Autodesk Fusion 360 part; units mm, degrees
(part 4 of 5)
sketch "Sketch14" plane through (0, -22.5, 0) normal (0, -1, 0) x (1, 0, 0)
  line L0 (26.575, -10) -> (26.575, 1)
  line L1 (26.575, 1) -> (-26.575, 1)
  line L2 (-26.575, 1) -> (-26.575, -10)
  line L3 (-26.575, -10) -> (26.575, -10)
  line L4 (-15.5, -1.5) -> (15.5, -1.5)
  line L5 (17.5, -3.5) -> (17.5, -5.5)
  line L6 (15.5, -7.5) -> (-15.5, -7.5)
  line L7 (-17.5, -5.5) -> (-17.5, -3.5)
  arc A0 (-15.5, -1.5) -> (-17.5, -3.5) centre (-15.5, -3.5) ccw
  arc A1 (-17.5, -5.5) -> (-15.5, -7.5) centre (-15.5, -5.5) ccw
  arc A2 (15.5, -7.5) -> (17.5, -5.5) centre (15.5, -5.5) ccw
  arc A3 (17.5, -3.5) -> (15.5, -1.5) centre (15.5, -3.5) ccw
  dimension "d131" = 2.5
  dimension "d132" = 2.5
  dimension "d133" = 9.075
  dimension "d134" = 9.075
  dimension "d135" = 2
  constraint horizontal L4
  constraint vertical L5
  constraint horizontal L6
  constraint vertical L7
  constraint tangent L4 A0
  constraint tangent L7 A0
  constraint tangent L7 A1
  constraint tangent L6 A1
  constraint equal A0 A1
  constraint tangent L6 A2
  constraint tangent L5 A2
  constraint equal A0 A2
  constraint tangent L4 A3
  constraint tangent L5 A3
  constraint equal A0 A3
  measures "d131" distance of L1 L4
  measures "d132" distance of L3 L6
  measures "d133" distance of L2 L7
  measures "d134" distance of L0 L5
  measures "d135" radius of A0
extrude "Extrude16" cut sketch "Sketch14" against normal blind 4 contours L4 L5 L6 L7 A0 A1 A2 A3 bodies 1
sketch "Sketch15" plane through (-26.575, 0, 0) normal (-1, 0, 0) x (0, -1, 0)
  line L0 (-22.5, 38.5) -> (-28.5, 38.5)
  line L1 (-28.5, 38.5) -> (-28.5, -10)
  line L2 (-28.5, -10) -> (22.5, -10)
  line L3 (22.5, -10) -> (22.5, 1)
  line L4 (22.5, 1) -> (-22.5, 1)
  line L5 (-22.5, 1) -> (-22.5, 38.5)
  line L6 (-13, -1.5) -> (13, -1.5)
  line L7 (15, -3.5) -> (15, -5.5)
  line L8 (13, -7.5) -> (-13, -7.5)
  line L9 (-15, -5.5) -> (-15, -3.5)
  arc A0 (15, -3.5) -> (13, -1.5) centre (13, -3.5) ccw
  arc A1 (13, -7.5) -> (15, -5.5) centre (13, -5.5) ccw
  arc A2 (-15, -5.5) -> (-13, -7.5) centre (-13, -5.5) ccw
  arc A3 (-13, -1.5) -> (-15, -3.5) centre (-13, -3.5) ccw
  dimension "d138" = 2.5
  dimension "d139" = 2.5
  dimension "d140" = 7.5
  dimension "d141" = 13.5
  dimension "d142" = 2
  constraint horizontal L6
  constraint vertical L7
  constraint horizontal L8
  constraint vertical L9
  constraint tangent L7 A0
  constraint tangent L6 A0
  constraint tangent L7 A1
  constraint tangent L8 A1
  constraint equal A0 A1
  constraint tangent L8 A2
  constraint tangent L9 A2
  constraint equal A0 A2
  constraint tangent L9 A3
  constraint tangent L6 A3
  constraint equal A0 A3
  measures "d138" distance of L4 L6
  measures "d139" distance of L2 L8
  measures "d140" distance of L3 L7
  measures "d141" distance of L1 L9
  measures "d142" radius of A0
extrude "Extrude17" cut sketch "Sketch15" against normal blind 4 contours L6 L7 L8 L9 A0 A1 A2 A3 bodies 1
sketch "Sketch16" plane through (0, 28.5, 0) normal (0, 1, 0) x (-1, 0, 0)
  line L0 (-24.075, 6) -> (-24.075, 7)
  arc A0 (-21.575, 9.5) -> (-24.075, 7) centre (-21.575, 7) ccw
  line L1 (-21.575, 9.5) -> (21.575, 9.5)
  arc A1 (24.075, 7) -> (21.575, 9.5) centre (21.575, 7) ccw
  line L2 (24.075, 7) -> (24.075, 6)
  arc A2 (21.575, 3.5) -> (24.075, 6) centre (21.575, 6) ccw
  line L3 (21.575, 3.5) -> (-21.575, 3.5)
  arc A3 (-24.075, 6) -> (-21.575, 3.5) centre (-21.575, 6) ccw
  circle A4 centre (0, 24.5) radius 12.5
  line L4 (26.575, 38.5) -> (-26.575, 38.5)
  line L5 (-26.575, 38.5) -> (-26.575, -10)
  line L6 (-26.575, -10) -> (26.575, -10)
  line L7 (26.575, -10) -> (26.575, 38.5)
  circle A5 centre (20, 18.5) radius 5
  circle A6 centre (-20, 30.5) radius 5
  circle A7 centre (20, 30.5) radius 5
  circle A8 centre (-20, 18.5) radius 5
  line L8 (-15.5, -1.5) -> (15.5, -1.5)
  line L9 (17.5, -3.5) -> (17.5, -5.5)
  line L10 (15.5, -7.5) -> (-15.5, -7.5)
  line L11 (-17.5, -5.5) -> (-17.5, -3.5)
  arc A9 (-15.5, -1.5) -> (-17.5, -3.5) centre (-15.5, -3.5) ccw
  arc A10 (-17.5, -5.5) -> (-15.5, -7.5) centre (-15.5, -5.5) ccw
  arc A11 (15.5, -7.5) -> (17.5, -5.5) centre (15.5, -5.5) ccw
  arc A12 (17.5, -3.5) -> (15.5, -1.5) centre (15.5, -3.5) ccw
  dimension "d145" = 5
  dimension "d146" = 2.5
  dimension "d147" = 9.075
  dimension "d148" = 9.075
  dimension "d149" = 2
  constraint horizontal L8
  constraint vertical L9
  constraint horizontal L10
  constraint vertical L11
  constraint tangent L8 A9
  constraint tangent L11 A9
  constraint tangent L11 A10
  constraint tangent L10 A10
  constraint equal A9 A10
  constraint tangent L10 A11
  constraint tangent L9 A11
  constraint equal A9 A11
  constraint tangent L9 A12
  constraint tangent L8 A12
  constraint equal A9 A12
  measures "d145" distance of L3 L8
  measures "d146" distance of L6 L10
  measures "d147" distance of L5 L11
  measures "d148" distance of L7 L9
  measures "d149" radius of A9
extrude "Extrude18" cut sketch "Sketch16" against normal blind 10 contours L8 L9 L10 L11 A9 A10 A11 A12 bodies 1
equation "d7 = ( 2.25 in / 2 )"
equation "d8 = ( 45 / 2 ) * 1 mm"
equation "d31 = ( 2.25 in - 40 mm ) / 2"
equation "d127 = 7.5 mm + 6 mm"
equation "d133 = ( ( 53.15 - 35 ) / 2 ) * 1 mm"
equation "d134 = ( ( 53.15 - 35 ) / 2 ) * 1 mm"

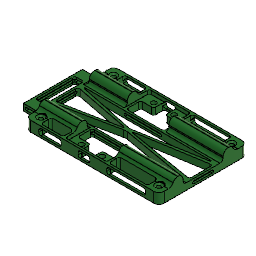
design "TM Foundation"
Autodesk Fusion 360 part; units mm, degrees
sketch "Sketch1" plane through (0, 0, 0) normal (0, 0, 1) x (1, 0, 0)
  line L0 (-72.5, 28.55) -> (72.5, 28.55)
  line L1 (72.5, 28.55) -> (72.5, -28.55)
  line L2 (72.5, -28.55) -> (-72.5, -28.55)
  line L3 (-72.5, -28.55) -> (-72.5, 28.55)
  dimension "d1" = 145
  dimension "d2" = 72.5
  dimension "d3" = 57.1
  dimension "d4" = 28.55
  constraint horizontal L0
  constraint vertical L1
  constraint horizontal L2
  constraint vertical L3
  measures "d1" distance of L1 L3
  measures "d2" distance of origin L1
  measures "d3" distance of L0 L2
  measures "d4" distance of origin L0
extrude "Extrude1" add sketch "Sketch1" along normal blind 6.5
ref_plane "WorkPlane1" through (-62.5, 0, 3.25) normal (-1, 0, 0) x (0, -1, 0)
sketch "Sketch6" plane through (-62.5, 0, 0) normal (-1, 0, 0) x (0, -1, 0)
  line L0 (-28.55, 6.5) -> (-28.55, 15.75)
  line L1 (-28.55, 15.75) -> (-24.3, 15.75)
  line L2 (-16.3, 6.5) -> (16.3, 6.5)
  line L3 (28.55, 6.5) -> (28.55, 15.75)
  line L4 (28.55, 15.75) -> (24.3, 15.75)
  line L5 (-19.3, 10.75) -> (-19.3, 9.5)
  line L6 (19.3, 10.75) -> (19.3, 9.5)
  arc A0 (-19.3, 9.5) -> (-16.3, 6.5) centre (-16.3, 9.5) ccw
  arc A1 (16.3, 6.5) -> (19.3, 9.5) centre (16.3, 9.5) ccw
  arc A2 (-19.3, 10.75) -> (-24.3, 15.75) centre (-24.3, 10.75) ccw
  arc A3 (24.3, 15.75) -> (19.3, 10.75) centre (24.3, 10.75) ccw
  line L7 (-28.55, 6.5) -> (28.55, 6.5)
  point P0 (-19.3, 15.75)
  point P1 (-28.55, 0)
  point P2 (-28.55, 6.5)
  point P3 (-28.55, 6.5)
  point P4 (19.3, 15.75)
  dimension "d36" = 9.25
  dimension "d37" = 9.25
  dimension "d38" = 57.1
  dimension "d39" = 9.25
  dimension "d40" = 9.25
  dimension "d41" = 3
  dimension "d42" = 5
  constraint vertical L0
  constraint perpendicular L0 L1
  constraint vertical P3 P1
  constraint coincident P3 P2
  constraint perpendicular L0 L2
  constraint perpendicular L2 L3
  constraint perpendicular L3 L4
  constraint perpendicular L2 L5
  constraint perpendicular L2 L6
  constraint coincident P3 L2
  constraint tangent L5 A0
  constraint tangent L2 A0
  constraint coincident L3.start L2
  constraint tangent L2 A1
  constraint tangent L6 A1
  constraint equal A0 A1
  constraint coincident P0 L1
  constraint coincident P0 L5
  constraint tangent L1 A2
  constraint tangent L5 A2
  constraint coincident P4 L6
  constraint coincident P4 L4
  constraint tangent L6 A3
  constraint tangent L4 A3
  constraint equal A2 A3
  measures "d36" distance of P3 L0.end
  measures "d37" distance of L0.end P0
  measures "d38" distance of P3 L3.start
  measures "d39" distance of L3.start L3.end
  measures "d40" distance of L3.end P4
  measures "d41" radius of A0
  measures "d42" radius of A2
extrude "Extrude6" add sketch "Sketch6" against normal blind 135
extrude "Extrude7" cut 2 faces at (-62.5, -24.05, 11) (-62.5, 24.05, 11) along direction (1, 0, 0) blind 6
extrude "Extrude12" add 1 faces at (29.5, -28.55, 7.4167) along direction (0, -1, 0) blind 14.05
extrude "Extrude13" add 1 faces at (29.5, 28.55, 7.4167) along direction (0, 1, 0) blind 14.05
sketch "Sketch10" plane through (0, 0, 15.75) normal (0, 0, 1) x (-1, 0, 0)
  line L0 (56.5, 24.3) -> (56.5, 42.6)
  line L1 (56.5, 42.6) -> (-72.5, 42.6)
  line L2 (-72.5, 42.6) -> (-72.5, 24.3)
  line L3 (-72.5, 24.3) -> (56.5, 24.3)
  line L4 (18.05, -40.6) -> (-18.05, -40.6)
  line L5 (-20.05, -38.6) -> (-20.05, 38.6)
  line L6 (-18.05, 40.6) -> (18.05, 40.6)
  line L7 (20.05, 38.6) -> (20.05, -38.6)
  line L8 (56.5, -42.6) -> (-72.5, -42.6)
  arc A0 (20.05, 38.6) -> (18.05, 40.6) centre (18.05, 38.6) ccw
  arc A1 (-18.05, 40.6) -> (-20.05, 38.6) centre (-18.05, 38.6) ccw
  arc A2 (-20.05, -38.6) -> (-18.05, -40.6) centre (-18.05, -38.6) ccw
  arc A3 (18.05, -40.6) -> (20.05, -38.6) centre (18.05, -38.6) ccw
  dimension "d68" = 52.45
  dimension "d69" = 36.45
  dimension "d70" = 2
  dimension "d71" = 2
  dimension "d74" = 2
  constraint horizontal L4
  constraint vertical L5
  constraint horizontal L6
  constraint vertical L7
  constraint tangent L7 A0
  constraint tangent L6 A0
  constraint tangent L6 A1
  constraint tangent L5 A1
  constraint equal A0 A1
  constraint tangent L5 A2
  constraint tangent L4 A2
  constraint equal A0 A2
  constraint tangent L4 A3
  constraint tangent L7 A3
  constraint equal A0 A3
  measures "d68" distance of L2 L5
  measures "d69" distance of L0 L7
  measures "d70" distance of L1 L6
  measures "d71" distance of L4 L8
  measures "d74" radius of A0
extrude "Extrude14" cut sketch "Sketch10" against normal blind 9.25 contours L3 L4 L5 L7 A2 A3 | L3 L5 L6 L7 A0 A1
sketch "Sketch11" plane through (0, 0, 6.5) normal (0, 0, 1) x (-1, 0, 0)
  line L0 (20.05, -16.3) -> (56.5, -16.3)
  line L1 (56.5, -16.3) -> (56.5, -42.6)
  line L2 (56.5, -42.6) -> (72.5, -42.6)
  line L3 (72.5, -42.6) -> (72.5, 42.6)
  line L4 (72.5, 42.6) -> (56.5, 42.6)
  line L5 (56.5, 42.6) -> (56.5, 16.3)
  line L6 (56.5, 16.3) -> (20.05, 16.3)
  line L7 (20.05, 16.3) -> (20.05, 38.6)
  arc A0 (20.05, 38.6) -> (18.05, 40.6) centre (18.05, 38.6) ccw
  line L8 (18.05, 40.6) -> (-18.05, 40.6)
  arc A1 (-18.05, 40.6) -> (-20.05, 38.6) centre (-18.05, 38.6) ccw
  line L9 (-20.05, 38.6) -> (-20.05, 16.3)
  line L10 (-20.05, 16.3) -> (-72.5, 16.3)
  line L11 (-72.5, 16.3) -> (-72.5, -16.3)
  line L12 (-72.5, -16.3) -> (-20.05, -16.3)
  line L13 (-20.05, -16.3) -> (-20.05, -38.6)
  arc A2 (-20.05, -38.6) -> (-18.05, -40.6) centre (-18.05, -38.6) ccw
  line L14 (-18.05, -40.6) -> (18.05, -40.6)
  arc A3 (18.05, -40.6) -> (20.05, -38.6) centre (18.05, -38.6) ccw
  line L15 (20.05, -38.6) -> (20.05, -16.3)
  point P0 (10, 34.75)
  point P1 (-10, 34.75)
  point P2 (-10, -34.75)
  point P3 (10, -34.75)
  dimension "d75" = 20
  dimension "d76" = 69.5
  dimension "d77" = 10.05
  dimension "d78" = 5.85
  constraint horizontal P2 P3
  constraint vertical P1 P2
  constraint horizontal P0 P1
  constraint vertical P0 P3
  measures "d75" distance of P0 P1
  measures "d76" distance of P1 P2
  measures "d77" distance of L7 P0
  measures "d78" distance of L8 P0
hole "Hole1" at (-10, 34.75, 6.5) at (10, 34.75, 6.5) at (10, -34.75, 6.5) at (-10, -34.75, 6.5) direction (0, 0, -1) diameter 4.85 end through all
sketch "Sketch12" plane through (0, 0, 6.5) normal (0, 0, 1) x (-1, 0, 0)
  circle A0 centre (-10, 34.75) radius 2.425
  circle A1 centre (10, -34.75) radius 2.425
  circle A2 centre (-10, -34.75) radius 2.425
  circle A3 centre (10, 34.75) radius 2.425
  line L0 (20.05, -16.3) -> (56.5, -16.3)
  line L1 (56.5, -16.3) -> (56.5, -42.6)
  line L2 (56.5, -42.6) -> (72.5, -42.6)
  line L3 (72.5, -42.6) -> (72.5, 42.6)
  line L4 (72.5, 42.6) -> (56.5, 42.6)
  line L5 (56.5, 42.6) -> (56.5, 16.3)
  line L6 (56.5, 16.3) -> (20.05, 16.3)
  line L7 (20.05, 16.3) -> (20.05, 38.6)
  arc A4 (20.05, 38.6) -> (18.05, 40.6) centre (18.05, 38.6) ccw
  line L8 (18.05, 40.6) -> (-18.05, 40.6)
  arc A5 (-18.05, 40.6) -> (-20.05, 38.6) centre (-18.05, 38.6) ccw
  line L9 (-20.05, 38.6) -> (-20.05, 16.3)
  line L10 (-20.05, 16.3) -> (-72.5, 16.3)
  line L11 (-72.5, 16.3) -> (-72.5, -16.3)
  line L12 (-72.5, -16.3) -> (-20.05, -16.3)
  line L13 (-20.05, -16.3) -> (-20.05, -38.6)
  arc A6 (-20.05, -38.6) -> (-18.05, -40.6) centre (-18.05, -38.6) ccw
  line L14 (-18.05, -40.6) -> (18.05, -40.6)
  arc A7 (18.05, -40.6) -> (20.05, -38.6) centre (18.05, -38.6) ccw
  line L15 (20.05, -38.6) -> (20.05, -16.3)
  line L16 (72.5, -42.6) -> (56.5, -42.6)
  line L17 (56.5, -42.6) -> (56.5, -28.5)
  line L18 (56.5, -28.5) -> (72.5, -28.5)
  line L19 (72.5, -28.5) -> (72.5, -42.6)
  line L20 (72.5, 42.6) -> (56.5, 42.6)
  line L21 (56.5, 42.6) -> (56.5, 28.5)
  line L22 (56.5, 28.5) -> (72.5, 28.5)
  line L23 (72.5, 28.5) -> (72.5, 42.6)
  dimension "d81" = 57
  dimension "d82" = 28.5
  constraint horizontal L16
  constraint vertical L17
  constraint horizontal L18
  constraint vertical L19
  constraint coincident L1 L17.end
  constraint coincident L2.end L3.start
  constraint horizontal L20
  constraint vertical L21
  constraint horizontal L22
  constraint vertical L23
  constraint coincident L5 L21.end
  constraint coincident L3.end L4.start
  measures "d81" distance of L18 L22
  measures "d82" distance of origin L22
extrude "Extrude15" cut sketch "Sketch12" against normal blind 6.5 contours L1 L2 L3 L16 L17 L18 L19 | L3 L4 L5 L20 L21 L22 L23
sketch "Sketch13" plane through (0, 0, 15.75) normal (0, 0, 1) x (-1, 0, 0)
  line L0 (20.05, 38.6) -> (20.05, 24.3)
  line L1 (20.05, 24.3) -> (56.5, 24.3)
  line L2 (56.5, 24.3) -> (56.5, 42.6)
  line L3 (56.5, 42.6) -> (-72.5, 42.6)
  line L4 (-72.5, 42.6) -> (-72.5, 24.3)
  line L5 (-72.5, 24.3) -> (-20.05, 24.3)
  line L6 (-20.05, 24.3) -> (-20.05, 38.6)
  arc A0 (-18.05, 40.6) -> (-20.05, 38.6) centre (-18.05, 38.6) ccw
  line L7 (-18.05, 40.6) -> (18.05, 40.6)
  arc A1 (20.05, 38.6) -> (18.05, 40.6) centre (18.05, 38.6) ccw
  line L8 (56.5, 42.6) -> (-72.5, 42.6)
  line L9 (-72.5, 42.6) -> (-72.5, 28.5)
  line L10 (-72.5, 28.5) -> (56.5, 28.5)
  line L11 (56.5, 28.5) -> (56.5, 42.6)
  line L12 (56.5, -42.6) -> (-72.5, -42.6)
  line L13 (-72.5, -42.6) -> (-72.5, -28.5)
  line L14 (-72.5, -28.5) -> (56.5, -28.5)
  line L15 (56.5, -28.5) -> (56.5, -42.6)
  line L16 (56.5, -28.5) -> (72.5, -28.5)
  dimension "d85" = 14.1
  dimension "d86" = 14.1
  dimension "d87" = 14.1
  constraint horizontal L8
  constraint vertical L9
  constraint horizontal L10
  constraint vertical L11
  constraint coincident L2.end L3.start
  constraint horizontal L12
  constraint vertical L13
  constraint horizontal L14
  constraint vertical L15
  constraint vertical L2.end L12.start
  constraint vertical L9.end L13.end
  constraint coincident L3.end L4.start
  measures "d85" distance of L8 L10
  measures "d86" distance of L12 L16
  measures "d87" distance of L12 L14
extrude "Extrude16" cut sketch "Sketch13" against normal blind 5.75 contours L0 L2 L3 L4 L6 A0 L7 A1 L8 L9 L10 L11 | L0 L6 A0 L7 A1 L10 | L12 L13 L14 L15
fillet "Fillet7" radius 5 8 edges at (-38.275, -28.5, 10) (-38.275, -28.5, 15.75) (46.275, -28.5, 10) (46.275, -28.5, 15.75) (-38.275, 28.5, 10) (-38.275, 28.5, 15.75) (46.275, 28.5, 10) (46.275, 28.5, 15.75)
fillet "Fillet8" radius 5 4 edges at (-56.5, -42.6, 5) (72.5, -42.6, 5) (72.5, 42.6, 5) (-56.5, 42.6, 5)
fillet "Fillet9" radius 5 2 edges at (-56.5, -28.5, 3.25) (-56.5, 28.5, 3.25)
fillet "Fillet10" radius 3 2 edges at (-56.5, 24.9, 6.5) (-56.5, -24.9, 6.5)
sketch "Sketch14" plane through (0, 0, 6.5) normal (0, 0, 1) x (-1, 0, 0)
  line L0 (59.5, 16.3) -> (20.05, 16.3)
  line L1 (20.05, 16.3) -> (20.05, 38.6)
  arc A0 (20.05, 38.6) -> (18.05, 40.6) centre (18.05, 38.6) ccw
  line L2 (18.05, 40.6) -> (-18.05, 40.6)
  arc A1 (-18.05, 40.6) -> (-20.05, 38.6) centre (-18.05, 38.6) ccw
  line L3 (-20.05, 38.6) -> (-20.05, 16.3)
  line L4 (-20.05, 16.3) -> (-72.5, 16.3)
  line L5 (-72.5, 16.3) -> (-72.5, -16.3)
  line L6 (-72.5, -16.3) -> (-20.05, -16.3)
  line L7 (-20.05, -16.3) -> (-20.05, -38.6)
  arc A2 (-20.05, -38.6) -> (-18.05, -40.6) centre (-18.05, -38.6) ccw
  line L8 (-18.05, -40.6) -> (18.05, -40.6)
  arc A3 (18.05, -40.6) -> (20.05, -38.6) centre (18.05, -38.6) ccw
  line L9 (20.05, -38.6) -> (20.05, -16.3)
  line L10 (20.05, -16.3) -> (59.5, -16.3)
  line L11 (59.5, -16.3) -> (59.5, -28.9174)
  arc A4 (61.5, -28.5) -> (59.5, -28.9174) centre (61.5, -33.5) ccw
  line L12 (61.5, -28.5) -> (72.5, -28.5)
  line L13 (72.5, -28.5) -> (72.5, 28.5)
  line L14 (72.5, 28.5) -> (61.5, 28.5)
  arc A5 (59.5, 28.9174) -> (61.5, 28.5) centre (61.5, 33.5) ccw
  line L15 (59.5, 28.9174) -> (59.5, 16.3)
  circle A6 centre (-10, 34.75) radius 2.425
  circle A7 centre (10, -34.75) radius 2.425
  circle A8 centre (-10, -34.75) radius 2.425
  circle A9 centre (10, 34.75) radius 2.425
  line L16 (68.5, -19) -> (63.5, -19)
  line L17 (61.5, -17) -> (61.5, 17)
  line L18 (63.5, 19) -> (68.5, 19)
  line L19 (70.5, 17) -> (70.5, -17)
  arc A10 (68.5, -19) -> (70.5, -17) centre (68.5, -17) ccw
  arc A11 (70.5, 17) -> (68.5, 19) centre (68.5, 17) ccw
  arc A12 (63.5, 19) -> (61.5, 17) centre (63.5, 17) ccw
  arc A13 (61.5, -17) -> (63.5, -19) centre (63.5, -17) ccw
  dimension "d100" = 2
  dimension "d101" = 2
  dimension "d104" = 2
  dimension "d285" = 9.5
  dimension "d286" = 9.5
  constraint horizontal L16
  constraint vertical L17
  constraint horizontal L18
  constraint vertical L19
  constraint tangent L16 A10
  constraint tangent L19 A10
  constraint tangent L19 A11
  constraint tangent L18 A11
  constraint equal A10 A11
  constraint tangent L18 A12
  constraint tangent L17 A12
  constraint equal A10 A12
  constraint tangent L17 A13
  constraint tangent L16 A13
  constraint equal A10 A13
  measures "d100" distance of L11 L17
  measures "d101" distance of L13 L19
  measures "d104" radius of A10
  measures "d285" distance of L14 L18
  measures "d286" distance of L12 L16
extrude "Extrude17" cut sketch "Sketch14" against normal blind 6.5 contours L16 L17 L18 L19 A10 A11 A12 A13
sketch "Sketch15" plane through (0, 0, 10) normal (0, 0, 1) x (-1, 0, 0)
  arc A0 (-67.5, 42.6) -> (-72.5, 37.6) centre (-67.5, 37.6) ccw
  line L0 (-72.5, 37.6) -> (-72.5, 33.5)
  line L1 (-72.5, 33.5) -> (-20.05, 33.5)
  line L2 (-20.05, 33.5) -> (-20.05, 38.6)
  arc A1 (-18.05, 40.6) -> (-20.05, 38.6) centre (-18.05, 38.6) ccw
  line L3 (-18.05, 40.6) -> (18.05, 40.6)
  arc A2 (20.05, 38.6) -> (18.05, 40.6) centre (18.05, 38.6) ccw
  line L4 (20.05, 38.6) -> (20.05, 33.5)
  line L5 (20.05, 33.5) -> (56.5, 33.5)
  line L6 (56.5, 33.5) -> (56.5, 37.6)
  arc A3 (56.5, 37.6) -> (51.5, 42.6) centre (51.5, 37.6) ccw
  line L7 (51.5, 42.6) -> (-67.5, 42.6)
  line L8 (51.5, -42.6) -> (-67.5, -42.6)
  line L9 (56.5, -33.5) -> (56.5, -37.6)
  point P0 (49, 35.1)
  point P1 (-65, 35.1)
  point P2 (-65, -35.1)
  point P3 (49, -35.1)
  dimension "d107" = 7.5
  dimension "d108" = 7.5
  dimension "d109" = 7.5
  dimension "d110" = 7.5
  constraint horizontal P2 P3
  constraint vertical P1 P2
  constraint horizontal P0 P1
  constraint vertical P0 P3
  measures "d107" distance of P3 L8
  measures "d108" distance of P3 L9
  measures "d109" distance of L0 P1
  measures "d110" distance of L7 P1
hole "Hole2" at (-49, 35.1, 10) at (65, 35.1, 10) at (65, -35.1, 10) at (-49, -35.1, 10) direction (0, 0, -1) diameter 3.797 end through all countersink diameter 7.087 countersink angle 100
sketch "Sketch17" plane through (0, 0, 10) normal (0, 0, 1) x (-1, 0, 0)
  arc A0 (-61.8383, 33.5) -> (-68.1617, 33.5) centre (-65, 35.1) ccw
  line L0 (-61.8383, 33.5) -> (-20.05, 33.5)
  line L1 (-20.05, 33.5) -> (-20.05, 38.6)
  arc A1 (-18.05, 40.6) -> (-20.05, 38.6) centre (-18.05, 38.6) ccw
  line L2 (-18.05, 40.6) -> (18.05, 40.6)
  arc A2 (20.05, 38.6) -> (18.05, 40.6) centre (18.05, 38.6) ccw
  line L3 (20.05, 38.6) -> (20.05, 33.5)
  line L4 (20.05, 33.5) -> (45.8383, 33.5)
  arc A3 (52.1617, 33.5) -> (45.8383, 33.5) centre (49, 35.1) ccw
  line L5 (52.1617, 33.5) -> (56.5, 33.5)
  line L6 (56.5, 33.5) -> (56.5, 37.6)
  arc A4 (56.5, 37.6) -> (51.5, 42.6) centre (51.5, 37.6) ccw
  line L7 (51.5, 42.6) -> (-67.5, 42.6)
  arc A5 (-67.5, 42.6) -> (-72.5, 37.6) centre (-67.5, 37.6) ccw
  line L8 (-72.5, 37.6) -> (-72.5, 33.5)
  line L9 (-72.5, 33.5) -> (-68.1617, 33.5)
  circle A6 centre (-65, 35.1) radius 4.25
  circle A7 centre (-65, -35.1) radius 4.25
  circle A8 centre (49, -35.1) radius 4.25
  circle A9 centre (49, 35.1) radius 1.8985
  circle A10 centre (49, 35.1) radius 4.25
  dimension "d124" = 8.5
  dimension "d125" = 8.5
  dimension "d126" = 70.2
  dimension "d127" = 8.5
  dimension "d130" = 8.5
  constraint concentric A0 A6
  constraint vertical A0.centre A7.centre
  constraint horizontal A7.centre A8.centre
  constraint concentric A3 A10
  measures "d124" diameter of A7
  measures "d125" diameter of A8
  measures "d126" distance of A8.centre A3.centre
  measures "d127" diameter of A6
  measures "d130" diameter of A10
extrude "Extrude19" cut sketch "Sketch17" along normal blind 2 contours A0 L0 L9 A6 | A0 L0 L9 A6 | L4 A3 L5 A10 | L4 A3 L5 A10 | A7 | A8 | A9
sketch "Sketch19" plane through (0, 0, 6.5) normal (0, 0, 1) x (-1, 0, 0)
  line L0 (61.5, -17) -> (61.5, 17)
  arc A0 (63.5, 19) -> (61.5, 17) centre (63.5, 17) ccw
  line L1 (63.5, 19) -> (68.5, 19)
  arc A1 (70.5, 17) -> (68.5, 19) centre (68.5, 17) ccw
  line L2 (70.5, 17) -> (70.5, -17)
  arc A2 (68.5, -19) -> (70.5, -17) centre (68.5, -17) ccw
  line L3 (68.5, -19) -> (63.5, -19)
  arc A3 (61.5, -17) -> (63.5, -19) centre (63.5, -17) ccw
  line L4 (59.5, 16.3) -> (20.05, 16.3)
  line L5 (20.05, 16.3) -> (20.05, 38.6)
  arc A4 (20.05, 38.6) -> (18.05, 40.6) centre (18.05, 38.6) ccw
  line L6 (18.05, 40.6) -> (-18.05, 40.6)
  arc A5 (-18.05, 40.6) -> (-20.05, 38.6) centre (-18.05, 38.6) ccw
  line L7 (-20.05, 38.6) -> (-20.05, 16.3)
  line L8 (-20.05, 16.3) -> (-72.5, 16.3)
  line L9 (-72.5, 16.3) -> (-72.5, -16.3)
  line L10 (-72.5, -16.3) -> (-20.05, -16.3)
  line L11 (-20.05, -16.3) -> (-20.05, -38.6)
  arc A6 (-20.05, -38.6) -> (-18.05, -40.6) centre (-18.05, -38.6) ccw
  line L12 (-18.05, -40.6) -> (18.05, -40.6)
  arc A7 (18.05, -40.6) -> (20.05, -38.6) centre (18.05, -38.6) ccw
  line L13 (20.05, -38.6) -> (20.05, -16.3)
  line L14 (20.05, -16.3) -> (59.5, -16.3)
  line L15 (59.5, -16.3) -> (59.5, -28.9174)
  arc A8 (61.5, -28.5) -> (59.5, -28.9174) centre (61.5, -33.5) ccw
  line L16 (61.5, -28.5) -> (72.5, -28.5)
  line L17 (72.5, -28.5) -> (72.5, 28.5)
  line L18 (72.5, 28.5) -> (61.5, 28.5)
  arc A9 (59.5, 28.9174) -> (61.5, 28.5) centre (61.5, 33.5) ccw
  line L19 (59.5, 28.9174) -> (59.5, 16.3)
  circle A10 centre (-10, 34.75) radius 2.425
  circle A11 centre (10, -34.75) radius 2.425
  circle A12 centre (-10, -34.75) radius 2.425
  circle A13 centre (10, 34.75) radius 2.425
  line L20 (59.5, -8.8707) -> (59.5, 8.8707)
  line L21 (-70.5, -8.9444) -> (-70.5, 8.9444)
  line L22 (55.628, -14.3) -> (-65.7592, -14.3)
  line L23 (55.628, 14.3) -> (-65.7592, 14.3)
  line L24 (55.7295, 13.3104) -> (1.8744, 2.1388)
  line L25 (-1.8855, 2.081) -> (-65.8457, 13.3075)
  line L26 (-68.1756, 10.918) -> (-4.7518, 0.4934)
  line L27 (-4.7518, -0.4934) -> (-68.1756, -10.918)
  line L28 (-65.8457, -13.3075) -> (-1.8855, -2.081)
  line L29 (1.8744, -2.1388) -> (55.7295, -13.3104)
  line L30 (57.1159, -10.8335) -> (4.2578, -0.4907)
  line L31 (4.2578, 0.4907) -> (57.1159, 10.8335)
  arc A14 (55.628, -14.3) -> (55.7295, -13.3104) centre (55.628, -13.8) ccw
  arc A15 (-65.8457, -13.3075) -> (-65.7592, -14.3) centre (-65.7592, -13.8) ccw
  arc A16 (-65.7592, 14.3) -> (-65.8457, 13.3075) centre (-65.7592, 13.8) ccw
  arc A17 (55.7295, 13.3104) -> (55.628, 14.3) centre (55.628, 13.8) ccw
  arc A18 (57.1159, -10.8335) -> (59.5, -8.8707) centre (57.5, -8.8707) ccw
  arc A19 (59.5, 8.8707) -> (57.1159, 10.8335) centre (57.5, 8.8707) ccw
  arc A20 (-68.1756, 10.918) -> (-70.5, 8.9444) centre (-68.5, 8.9444) ccw
  arc A21 (-70.5, -8.9444) -> (-68.1756, -10.918) centre (-68.5, -8.9444) ccw
  arc A22 (-1.8855, 2.081) -> (1.8744, 2.1388) centre (-0.1567, 11.9304) ccw
  arc A23 (1.8744, -2.1388) -> (-1.8855, -2.081) centre (-0.1567, -11.9304) ccw
  arc A24 (-4.7518, -0.4934) -> (-4.7518, 0.4934) centre (-4.8329, 0) ccw
  arc A25 (4.2578, 0.4907) -> (4.2578, -0.4907) centre (4.3538, 0) ccw
  point P0 (-70.5, -11.3)
  point P1 (-70.5, 11.3)
  point P2 (60.5, 14.3)
  point P3 (-71.5, 14.3)
  point P4 (0, 1.75)
  point P5 (-1.75, 0)
  point P6 (0, -1.75)
  point P7 (1.75, 0)
  dimension "d143" = 2
  dimension "d144" = 2
  dimension "d145" = 5
  dimension "d146" = 5
  dimension "d147" = 2
  dimension "d148" = 2
  dimension "d149" = 1
  dimension "d150" = 1
  dimension "d151" = 3.5
  dimension "d152" = 3.5
  dimension "d153" = 1.75
  dimension "d154" = 1.75
  dimension "d155" = 0.5
  dimension "d156" = 2
  dimension "d157" = 10
  dimension "d158" = 0.5
  constraint perpendicular L14 L20
  constraint perpendicular L8 L21
  constraint perpendicular L15 L22
  constraint perpendicular L21 L23
  constraint vertical P4 P6
  constraint vertical origin P4
  constraint horizontal P5 P7
  constraint horizontal origin P7
  constraint tangent L22 A14
  constraint tangent L29 A14
  constraint tangent L28 A15
  constraint tangent L22 A15
  constraint equal A14 A15
  constraint coincident P3 L25
  constraint coincident P3 L23
  constraint tangent L25 A16
  constraint tangent L23 A16
  constraint equal A14 A16
  constraint coincident P2 L23
  constraint coincident P2 L24
  constraint tangent L23 A17
  constraint tangent L24 A17
  constraint equal A14 A17
  constraint tangent L30 A18
  constraint tangent L20 A18
  constraint tangent L20 A19
  constraint tangent L31 A19
  constraint equal A18 A19
  constraint coincident P1 L26
  constraint coincident P1 L21
  constraint tangent L26 A20
  constraint tangent L21 A20
  constraint equal A18 A20
  constraint coincident P0 L21
  constraint coincident P0 L27
  constraint tangent L21 A21
  constraint tangent L27 A21
  constraint equal A18 A21
  constraint tangent L24 A22
  constraint tangent L25 A22
  constraint tangent L29 A23
  constraint tangent L28 A23
  constraint equal A22 A23
  constraint tangent L27 A24
  constraint tangent L26 A24
  constraint tangent L31 A25
  constraint tangent L30 A25
  constraint equal A24 A25
  measures "d143" distance of L0 L20
  measures "d144" distance of L9 L21
  measures "d145" distance of L10 P0
  measures "d146" distance of L8 P1
  measures "d147" distance of L4 L23
  measures "d148" distance of L14 L22
  measures "d149" distance of L9 P3
  measures "d150" distance of L0 P2
  measures "d151" distance of P4 P6
  measures "d152" distance of P5 P7
  measures "d153" distance of origin P4
  measures "d154" distance of origin P5
  measures "d155" radius of A14
  measures "d157" radius of A22
  measures "d158" radius of A24
extrude "Extrude21" cut sketch "Sketch19" against normal blind 6.5 contours L20 L30 L31 A18 A19 A25 | L21 L26 L27 A20 A21 A24 | L22 L28 L29 A14 A15 A23 | L23 L24 L25 A16 A17 A22
sketch "Sketch20" plane through (0, 0, 6.5) normal (0, 0, 1) x (-1, 0, 0)
  line L0 (-4.7518, -0.4934) -> (-68.1756, -10.918)
  arc A0 (-70.5, -8.9444) -> (-68.1756, -10.918) centre (-68.5, -8.9444) ccw
  line L1 (-70.5, -8.9444) -> (-70.5, 8.9444)
  arc A1 (-68.1756, 10.918) -> (-70.5, 8.9444) centre (-68.5, 8.9444) ccw
  line L2 (-68.1756, 10.918) -> (-4.7518, 0.4934)
  arc A2 (-4.7518, -0.4934) -> (-4.7518, 0.4934) centre (-4.8329, 0) ccw
  line L3 (59.5, 8.8707) -> (59.5, -8.8707)
  arc A3 (57.1159, -10.8335) -> (59.5, -8.8707) centre (57.5, -8.8707) ccw
  line L4 (57.1159, -10.8335) -> (4.2578, -0.4907)
  arc A4 (4.2578, 0.4907) -> (4.2578, -0.4907) centre (4.3538, 0) ccw
  line L5 (4.2578, 0.4907) -> (57.1159, 10.8335)
  arc A5 (59.5, 8.8707) -> (57.1159, 10.8335) centre (57.5, 8.8707) ccw
  line L6 (-65.7592, 14.3) -> (55.628, 14.3)
  arc A6 (55.7295, 13.3104) -> (55.628, 14.3) centre (55.628, 13.8) ccw
  line L7 (55.7295, 13.3104) -> (1.8744, 2.1388)
  arc A7 (-1.8855, 2.081) -> (1.8744, 2.1388) centre (-0.1567, 11.9304) ccw
  line L8 (-1.8855, 2.081) -> (-65.8457, 13.3075)
  arc A8 (-65.7592, 14.3) -> (-65.8457, 13.3075) centre (-65.7592, 13.8) ccw
  line L9 (1.8744, -2.1388) -> (55.7295, -13.3104)
  arc A9 (55.628, -14.3) -> (55.7295, -13.3104) centre (55.628, -13.8) ccw
  line L10 (55.628, -14.3) -> (-65.7592, -14.3)
  arc A10 (-65.8457, -13.3075) -> (-65.7592, -14.3) centre (-65.7592, -13.8) ccw
  line L11 (-65.8457, -13.3075) -> (-1.8855, -2.081)
  arc A11 (1.8744, -2.1388) -> (-1.8855, -2.081) centre (-0.1567, -11.9304) ccw
  line L12 (61.5, -17) -> (61.5, 17)
  arc A12 (63.5, 19) -> (61.5, 17) centre (63.5, 17) ccw
  line L13 (63.5, 19) -> (68.5, 19)
  arc A13 (70.5, 17) -> (68.5, 19) centre (68.5, 17) ccw
  line L14 (70.5, 17) -> (70.5, -17)
  arc A14 (68.5, -19) -> (70.5, -17) centre (68.5, -17) ccw
  line L15 (68.5, -19) -> (63.5, -19)
  arc A15 (61.5, -17) -> (63.5, -19) centre (63.5, -17) ccw
  line L16 (59.5, 16.3) -> (20.05, 16.3)
  line L17 (20.05, 16.3) -> (20.05, 38.6)
  arc A16 (20.05, 38.6) -> (18.05, 40.6) centre (18.05, 38.6) ccw
  line L18 (18.05, 40.6) -> (-18.05, 40.6)
  arc A17 (-18.05, 40.6) -> (-20.05, 38.6) centre (-18.05, 38.6) ccw
  line L19 (-20.05, 38.6) -> (-20.05, 16.3)
  line L20 (-20.05, 16.3) -> (-72.5, 16.3)
  line L21 (-72.5, 16.3) -> (-72.5, -16.3)
  line L22 (-72.5, -16.3) -> (-20.05, -16.3)
  line L23 (-20.05, -16.3) -> (-20.05, -38.6)
  arc A18 (-20.05, -38.6) -> (-18.05, -40.6) centre (-18.05, -38.6) ccw
  line L24 (-18.05, -40.6) -> (18.05, -40.6)
  arc A19 (18.05, -40.6) -> (20.05, -38.6) centre (18.05, -38.6) ccw
  line L25 (20.05, -38.6) -> (20.05, -16.3)
  line L26 (20.05, -16.3) -> (59.5, -16.3)
  line L27 (59.5, -16.3) -> (59.5, -28.9174)
  arc A20 (61.5, -28.5) -> (59.5, -28.9174) centre (61.5, -33.5) ccw
  line L28 (61.5, -28.5) -> (72.5, -28.5)
  line L29 (72.5, -28.5) -> (72.5, 28.5)
  line L30 (72.5, 28.5) -> (61.5, 28.5)
  arc A21 (59.5, 28.9174) -> (61.5, 28.5) centre (61.5, 33.5) ccw
  line L31 (59.5, 28.9174) -> (59.5, 16.3)
  circle A22 centre (-10, 34.75) radius 2.425
  circle A23 centre (10, -34.75) radius 2.425
  circle A24 centre (-10, -34.75) radius 2.425
  circle A25 centre (10, 34.75) radius 2.425
  line L32 (16.05, 16.3) -> (-16.05, 16.3)
  line L33 (-18.05, 18.3) -> (-18.05, 28.325)
  line L34 (-16.05, 30.325) -> (-7.575, 30.325)
  line L35 (18.05, 28.325) -> (18.05, 18.3)
  line L36 (-7.575, -30.325) -> (-16.05, -30.325)
  line L37 (-18.05, -28.325) -> (-18.05, -18.3)
  line L38 (-16.05, -16.3) -> (16.05, -16.3)
  line L39 (18.05, -18.3) -> (18.05, -28.325)
  arc A26 (16.05, 16.3) -> (18.05, 18.3) centre (16.05, 18.3) ccw
  arc A27 (18.05, 28.325) -> (16.05, 30.325) centre (16.05, 28.325) ccw
  arc A28 (-16.05, 30.325) -> (-18.05, 28.325) centre (-16.05, 28.325) ccw
  arc A29 (-18.05, 18.3) -> (-16.05, 16.3) centre (-16.05, 18.3) ccw
  arc A30 (18.05, -18.3) -> (16.05, -16.3) centre (16.05, -18.3) ccw
  arc A31 (16.05, -30.325) -> (18.05, -28.325) centre (16.05, -28.325) ccw
  arc A32 (-18.05, -28.325) -> (-16.05, -30.325) centre (-16.05, -28.325) ccw
  arc A33 (-16.05, -16.3) -> (-18.05, -18.3) centre (-16.05, -18.3) ccw
  line L40 (5.575, -32.325) -> (5.575, -38.6)
  line L41 (3.575, -40.6) -> (-3.575, -40.6)
  line L42 (-5.575, -38.6) -> (-5.575, -32.325)
  arc A34 (-5.575, -32.325) -> (-7.575, -30.325) centre (-7.575, -32.325) ccw
  line L43 (16.05, -30.325) -> (7.575, -30.325)
  arc A35 (7.575, -30.325) -> (5.575, -32.325) centre (7.575, -32.325) ccw
  arc A36 (-5.575, -38.6) -> (-3.575, -40.6) centre (-3.575, -38.6) ccw
  arc A37 (3.575, -40.6) -> (5.575, -38.6) centre (3.575, -38.6) ccw
  line L44 (-5.575, 30.325) -> (5.575, 30.325)
  line L45 (5.575, 32.325) -> (5.575, 38.6)
  line L46 (3.575, 40.6) -> (-3.575, 40.6)
  line L47 (-5.575, 38.6) -> (-5.575, 32.325)
  arc A38 (-3.575, 40.6) -> (-5.575, 38.6) centre (-3.575, 38.6) ccw
  arc A39 (5.575, 38.6) -> (3.575, 40.6) centre (3.575, 38.6) ccw
  arc A40 (-7.575, 30.325) -> (-5.575, 32.325) centre (-7.575, 32.325) ccw
  line L48 (7.575, 30.325) -> (16.05, 30.325)
  arc A41 (5.575, 32.325) -> (7.575, 30.325) centre (7.575, 32.325) ccw
  line L49 (-67.5, 42.6) -> (51.5, 42.6)
  line L50 (51.5, -42.6) -> (-67.5, -42.6)
  dimension "d161" = 4.425
  dimension "d162" = 4.425
  dimension "d163" = 2
  dimension "d164" = 2
  dimension "d165" = 2
  dimension "d166" = 2
  dimension "d167" = 2
  dimension "d168" = 2
  dimension "d215" = 4.425
  dimension "d216" = 4.425
  dimension "d218" = 2
  dimension "d219" = 2
  dimension "d220" = 2
  dimension "d221" = 4.425
  dimension "d222" = 4.425
  dimension "d224" = 2
  dimension "d225" = 2
  dimension "d226" = 2
  dimension "d254" = 2
  dimension "d255" = 2
  constraint horizontal L32
  constraint vertical L33
  constraint horizontal L34
  constraint vertical L35
  constraint horizontal L36
  constraint vertical L37
  constraint horizontal L38
  constraint vertical L39
  constraint tangent L32 A26
  constraint tangent L35 A26
  constraint tangent L35 A27
  constraint tangent L34 A27
  constraint equal A26 A27
  constraint tangent L34 A28
  constraint tangent L33 A28
  constraint equal A26 A28
  constraint tangent L33 A29
  constraint tangent L32 A29
  constraint equal A26 A29
  constraint tangent L38 A30
  constraint tangent L39 A30
  constraint tangent L39 A31
  constraint tangent L36 A31
  constraint equal A30 A31
  constraint tangent L36 A32
  constraint tangent L37 A32
  constraint equal A30 A32
  constraint tangent L37 A33
  constraint tangent L38 A33
  constraint equal A30 A33
  constraint vertical L40
  constraint horizontal L41
  constraint vertical L42
  constraint coincident L36 A31.start
  constraint tangent L42 A34
  constraint tangent L36 A34
  constraint tangent A31 L43
  constraint tangent L40 A35
  constraint tangent L43 A35
  constraint tangent L42 A36
  constraint tangent L41 A36
  constraint tangent L41 A37
  constraint tangent L40 A37
  constraint equal A36 A37
  constraint horizontal L44
  constraint vertical L45
  constraint horizontal L46
  constraint vertical L47
  constraint coincident L34 L44.start
  constraint tangent L47 A38
  constraint tangent L46 A38
  constraint tangent L46 A39
  constraint tangent L45 A39
  constraint equal A38 A39
  constraint coincident L44.start L47
  constraint tangent L47 A40
  constraint tangent L34 A40
  constraint tangent A27 L48
  constraint coincident L44.end L45
  constraint coincident L44.end L48
  constraint tangent L45 A41
  constraint tangent L48 A41
  measures "d161" distance of A25.centre L34
  measures "d162" distance of A23.centre L36
  measures "d163" distance of L25 L39
  measures "d164" distance of L23 L37
  measures "d165" distance of L6 L32
  measures "d166" distance of L10 L38
  measures "d167" radius of A26
  measures "d168" radius of A30
  measures "d215" distance of A23.centre L40
  measures "d216" distance of A24.centre L42
  measures "d218" radius of A34
  measures "d219" radius of A35
  measures "d220" radius of A36
  measures "d221" distance of A25.centre L45
  measures "d222" distance of A22.centre L47
  measures "d224" radius of A38
  measures "d225" radius of A40
  measures "d226" radius of A41
  measures "d254" distance of L46 L49
  measures "d255" distance of L41 L50
extrude "Extrude22" cut sketch "Sketch20" against normal blind 6.5 contours L18 L32 L33 L34 L35 A26 A27 A28 A29 L45 L46 L47 A38 A39 A40 L48 A41 | L24 L36 L37 L38 L39 A30 A31 A32 A33 L40 L41 L42 A34 L43 A35 A36 A37
ref_plane "WorkPlane3" through (8, -36.725, 15) normal (0, 0, 1) x (1, 0, 0)
sketch "Sketch21" plane through (0, 0, 15) normal (0, 0, 1) x (1, 0, 0)
  line L0 (-41.4565, -30.974) -> (-24.05, -30.974)
  line L1 (-22.05, -32.974) -> (-22.05, -38.6)
  line L2 (-24.05, -40.6) -> (-41.4565, -40.6)
  line L3 (-43.4565, -38.6) -> (-43.4565, -32.974)
  line L4 (24.05, -30.974) -> (57.4565, -30.974)
  line L5 (59.4565, -32.974) -> (59.4565, -38.6)
  line L6 (57.4565, -40.6) -> (24.05, -40.6)
  line L7 (22.05, -38.6) -> (22.05, -32.974)
  line L8 (-41.4565, 40.6) -> (-24.05, 40.6)
  line L9 (-22.05, 38.6) -> (-22.05, 32.974)
  line L10 (-24.05, 30.974) -> (-41.4565, 30.974)
  line L11 (-43.4565, 32.974) -> (-43.4565, 38.6)
  line L12 (24.05, 40.6) -> (57.4565, 40.6)
  line L13 (59.4565, 38.6) -> (59.4565, 32.974)
  line L14 (57.4565, 30.974) -> (24.05, 30.974)
  line L15 (22.05, 32.974) -> (22.05, 38.6)
  line L16 (67.5, -42.6) -> (-51.5, -42.6)
  line L17 (-51.5, 42.6) -> (67.5, 42.6)
  line L18 (-20.05, -33.5) -> (-20.05, -38.6)
  line L19 (20.05, 33.5) -> (20.05, 38.6)
  line L20 (-56.5, -28.974) -> (-20.05, -28.974)
  line L21 (-20.05, 28.974) -> (-56.5, 28.974)
  circle A0 centre (-49, -35.1) radius 3.5435
  circle A1 centre (65, 35.1) radius 3.5435
  arc A2 (-41.4565, 40.6) -> (-43.4565, 38.6) centre (-41.4565, 38.6) ccw
  arc A3 (-22.05, 38.6) -> (-24.05, 40.6) centre (-24.05, 38.6) ccw
  arc A4 (-24.05, 30.974) -> (-22.05, 32.974) centre (-24.05, 32.974) ccw
  arc A5 (-43.4565, 32.974) -> (-41.4565, 30.974) centre (-41.4565, 32.974) ccw
  arc A6 (24.05, 40.6) -> (22.05, 38.6) centre (24.05, 38.6) ccw
  arc A7 (59.4565, 38.6) -> (57.4565, 40.6) centre (57.4565, 38.6) ccw
  arc A8 (57.4565, 30.974) -> (59.4565, 32.974) centre (57.4565, 32.974) ccw
  arc A9 (22.05, 32.974) -> (24.05, 30.974) centre (24.05, 32.974) ccw
  arc A10 (-41.4565, -30.974) -> (-43.4565, -32.974) centre (-41.4565, -32.974) ccw
  arc A11 (-22.05, -32.974) -> (-24.05, -30.974) centre (-24.05, -32.974) ccw
  arc A12 (-24.05, -40.6) -> (-22.05, -38.6) centre (-24.05, -38.6) ccw
  arc A13 (-43.4565, -38.6) -> (-41.4565, -40.6) centre (-41.4565, -38.6) ccw
  arc A14 (24.05, -30.974) -> (22.05, -32.974) centre (24.05, -32.974) ccw
  arc A15 (59.4565, -32.974) -> (57.4565, -30.974) centre (57.4565, -32.974) ccw
  arc A16 (57.4565, -40.6) -> (59.4565, -38.6) centre (57.4565, -38.6) ccw
  arc A17 (22.05, -38.6) -> (24.05, -40.6) centre (24.05, -38.6) ccw
  dimension "d172" = 2
  dimension "d173" = 2
  dimension "d174" = 2
  dimension "d175" = 2
  dimension "d176" = 2
  dimension "d177" = 2
  dimension "d178" = 5.5435
  dimension "d179" = 5.5435
  dimension "d180" = 2
  dimension "d181" = 2
  dimension "d182" = 2
  dimension "d183" = 2
  constraint horizontal L0
  constraint vertical L1
  constraint horizontal L2
  constraint vertical L3
  constraint horizontal L4
  constraint vertical L5
  constraint horizontal L6
  constraint vertical L7
  constraint horizontal L8
  constraint vertical L9
  constraint horizontal L10
  constraint vertical L11
  constraint horizontal L12
  constraint vertical L13
  constraint horizontal L14
  constraint vertical L15
  constraint tangent L8 A2
  constraint tangent L11 A2
  constraint tangent L8 A3
  constraint tangent L9 A3
  constraint equal A2 A3
  constraint tangent L9 A4
  constraint tangent L10 A4
  constraint equal A2 A4
  constraint tangent L10 A5
  constraint tangent L11 A5
  constraint equal A2 A5
  constraint tangent L15 A6
  constraint tangent L12 A6
  constraint tangent L12 A7
  constraint tangent L13 A7
  constraint equal A6 A7
  constraint tangent L13 A8
  constraint tangent L14 A8
  constraint equal A6 A8
  constraint tangent L14 A9
  constraint tangent L15 A9
  constraint equal A6 A9
  constraint tangent L3 A10
  constraint tangent L0 A10
  constraint tangent L0 A11
  constraint tangent L1 A11
  constraint equal A10 A11
  constraint tangent L1 A12
  constraint tangent L2 A12
  constraint equal A10 A12
  constraint tangent L2 A13
  constraint tangent L3 A13
  constraint equal A10 A13
  constraint tangent L7 A14
  constraint tangent L4 A14
  constraint tangent L4 A15
  constraint tangent L5 A15
  constraint equal A14 A15
  constraint tangent L5 A16
  constraint tangent L6 A16
  constraint equal A14 A16
  constraint tangent L6 A17
  constraint tangent L7 A17
  constraint equal A14 A17
  constraint vertical A8.centre A15.centre
  constraint vertical A9.centre A14.centre
  constraint horizontal A11.centre A14.centre
  constraint horizontal A12.centre A17.centre
  constraint vertical A4.centre A11.centre
  constraint vertical A5.centre A10.centre
  constraint horizontal A4.centre A9.centre
  constraint horizontal A3.centre A6.centre
  measures "d172" distance of L2 L16
  measures "d173" distance of L8 L17
  measures "d174" distance of L1 L18
  measures "d175" distance of L15 L19
  measures "d176" distance of L0 L20
  measures "d177" distance of L10 L21
  measures "d178" distance of L3 A0.centre
  measures "d179" distance of L13 A1.centre
  measures "d180" radius of A2
  measures "d181" radius of A6
  measures "d182" radius of A10
  measures "d183" radius of A14
extrude "Extrude23" cut sketch "Sketch21" against normal blind 15 contours L0 L1 L2 L3 A10 A11 A12 A13 | L4 L5 L6 L7 A14 A15 A16 A17 | L8 L9 L10 L11 A2 A3 A4 A5 | L12 L13 L14 L15 A6 A7 A8 A9
sketch "Sketch22" plane through (-72.5, 0, 0) normal (-1, 0, 0) x (0, -1, 0)
  line L0 (-28.5, 6.5) -> (-28.5, 0)
  line L1 (-28.5, 0) -> (28.5, 0)
  line L2 (28.5, 0) -> (28.5, 6.5)
  line L3 (28.5, 6.5) -> (-28.5, 6.5)
  line L4 (-18, 4.5) -> (18, 4.5)
  line L5 (19, 3.5) -> (19, 3)
  line L6 (18, 2) -> (-18, 2)
  line L7 (-19, 3) -> (-19, 3.5)
  arc A0 (-18, 4.5) -> (-19, 3.5) centre (-18, 3.5) ccw
  arc A1 (-19, 3) -> (-18, 2) centre (-18, 3) ccw
  arc A2 (18, 2) -> (19, 3) centre (18, 3) ccw
  arc A3 (19, 3.5) -> (18, 4.5) centre (18, 3.5) ccw
  dimension "d186" = 2
  dimension "d187" = 2
  dimension "d190" = 1
  dimension "d287" = 9.5
  dimension "d288" = 9.5
  constraint horizontal L4
  constraint vertical L5
  constraint horizontal L6
  constraint vertical L7
  constraint tangent L4 A0
  constraint tangent L7 A0
  constraint tangent L7 A1
  constraint tangent L6 A1
  constraint equal A0 A1
  constraint tangent L6 A2
  constraint tangent L5 A2
  constraint equal A0 A2
  constraint tangent L5 A3
  constraint tangent L4 A3
  constraint equal A0 A3
  measures "d186" distance of L3 L4
  measures "d187" distance of L1 L6
  measures "d190" radius of A0
  measures "d287" distance of L2 L5
  measures "d288" distance of L0 L7
extrude "Extrude24" cut sketch "Sketch22" against normal blind 5 contours L4 L5 L6 L7 A0 A1 A2 A3
sketch "Sketch23" plane through (-61.5, 0, 0) normal (-1, 0, 0) x (0, -1, 0)
  line L0 (17, 6.5) -> (-17, 6.5)
  line L1 (-17, 6.5) -> (-17, 0)
  line L2 (-17, 0) -> (17, 0)
  line L3 (17, 0) -> (17, 6.5)
  line L4 (-9, 4.5) -> (9, 4.5)
  line L5 (10, 3.5) -> (10, 3)
  line L6 (9, 2) -> (-9, 2)
  line L7 (-10, 3) -> (-10, 3.5)
  arc A0 (-9, 4.5) -> (-10, 3.5) centre (-9, 3.5) ccw
  arc A1 (-10, 3) -> (-9, 2) centre (-9, 3) ccw
  arc A2 (9, 2) -> (10, 3) centre (9, 3) ccw
  arc A3 (10, 3.5) -> (9, 4.5) centre (9, 3.5) ccw
  dimension "d193" = 20
  dimension "d194" = 10
  dimension "d195" = 2
  dimension "d196" = 2
  dimension "d197" = 1
  constraint horizontal L4
  constraint vertical L5
  constraint horizontal L6
  constraint vertical L7
  constraint tangent L4 A0
  constraint tangent L7 A0
  constraint tangent L7 A1
  constraint tangent L6 A1
  constraint equal A0 A1
  constraint tangent L6 A2
  constraint tangent L5 A2
  constraint equal A0 A2
  constraint tangent L5 A3
  constraint tangent L4 A3
  constraint equal A0 A3
  measures "d193" distance of L5 L7
  measures "d194" distance of origin L7
  measures "d195" distance of L2 L6
  measures "d196" distance of L0 L4
  measures "d197" radius of A0
extrude "Extrude25" cut sketch "Sketch23" against normal blind 5 contours L4 L5 L6 L7 A0 A1 A2 A3
sketch "Sketch24" plane through (72.5, 0, 0) normal (1, 0, 0) x (0, 1, 0)
  line L0 (37.6, 0) -> (37.6, 10)
  line L1 (37.6, 10) -> (33.5, 10)
  arc A0 (28.974, 12.875) -> (33.5, 10) centre (33.5, 15) ccw
  arc A1 (28.974, 12.875) -> (24.4481, 15.75) centre (24.4481, 10.75) ccw
  line L2 (24.4481, 15.75) -> (24.3, 15.75)
  arc A2 (24.3, 15.75) -> (19.3, 10.75) centre (24.3, 10.75) ccw
  line L3 (19.3, 10.75) -> (19.3, 9.5)
  arc A3 (16.3, 6.5) -> (19.3, 9.5) centre (16.3, 9.5) ccw
  line L4 (16.3, 6.5) -> (-16.3, 6.5)
  arc A4 (-19.3, 9.5) -> (-16.3, 6.5) centre (-16.3, 9.5) ccw
  line L5 (-19.3, 9.5) -> (-19.3, 10.75)
  arc A5 (-19.3, 10.75) -> (-24.3, 15.75) centre (-24.3, 10.75) ccw
  line L6 (-24.3, 15.75) -> (-24.4481, 15.75)
  arc A6 (-24.4481, 15.75) -> (-28.974, 12.875) centre (-24.4481, 10.75) ccw
  arc A7 (-33.5, 10) -> (-28.974, 12.875) centre (-33.5, 15) ccw
  line L7 (-33.5, 10) -> (-37.6, 10)
  line L8 (-37.6, 10) -> (-37.6, 0)
  line L9 (-37.6, 0) -> (37.6, 0)
  line L10 (-9, 4.5) -> (9, 4.5)
  line L11 (10, 3.5) -> (10, 3)
  line L12 (9, 2) -> (-9, 2)
  line L13 (-10, 3) -> (-10, 3.5)
  arc A8 (-9, 4.5) -> (-10, 3.5) centre (-9, 3.5) ccw
  arc A9 (-10, 3) -> (-9, 2) centre (-9, 3) ccw
  arc A10 (9, 2) -> (10, 3) centre (9, 3) ccw
  arc A11 (10, 3.5) -> (9, 4.5) centre (9, 3.5) ccw
  dimension "d200" = 2
  dimension "d201" = 2
  dimension "d202" = 10
  dimension "d203" = 20
  dimension "d204" = 1
  constraint horizontal L10
  constraint vertical L11
  constraint horizontal L12
  constraint vertical L13
  constraint tangent L10 A8
  constraint tangent L13 A8
  constraint tangent L13 A9
  constraint tangent L12 A9
  constraint equal A8 A9
  constraint tangent L12 A10
  constraint tangent L11 A10
  constraint equal A8 A10
  constraint tangent L11 A11
  constraint tangent L10 A11
  constraint equal A8 A11
  measures "d200" distance of L4 L10
  measures "d201" distance of L9 L12
  measures "d202" distance of origin L11
  measures "d203" distance of L11 L13
  measures "d204" radius of A8
extrude "Extrude26" cut sketch "Sketch24" against normal blind 5 contours L10 L11 L12 L13 A8 A9 A10 A11
sketch "Sketch25" plane through (0, 14.3, 0) normal (0, -1, 0) x (1, 0, 0)
  line L0 (65.7592, 6.5) -> (-55.628, 6.5)
  line L1 (-55.628, 6.5) -> (-55.628, 0)
  line L2 (-55.628, 0) -> (65.7592, 0)
  line L3 (65.7592, 0) -> (65.7592, 6.5)
  line L4 (-17.05, 4.5) -> (17.05, 4.5)
  line L5 (18.05, 3.5) -> (18.05, 3)
  line L6 (17.05, 2) -> (-17.05, 2)
  line L7 (-18.05, 3) -> (-18.05, 3.5)
  line L8 (67.5, 10) -> (-51.5, 10)
  arc A0 (-17.05, 4.5) -> (-18.05, 3.5) centre (-17.05, 3.5) ccw
  arc A1 (-18.05, 3) -> (-17.05, 2) centre (-17.05, 3) ccw
  arc A2 (17.05, 2) -> (18.05, 3) centre (17.05, 3) ccw
  arc A3 (18.05, 3.5) -> (17.05, 4.5) centre (17.05, 3.5) ccw
  dimension "d207" = 36.1
  dimension "d208" = 18.05
  dimension "d209" = 2
  dimension "d211" = 1
  dimension "d212" = 2
  constraint horizontal L4
  constraint vertical L5
  constraint horizontal L6
  constraint vertical L7
  constraint tangent L4 A0
  constraint tangent L7 A0
  constraint tangent L7 A1
  constraint tangent L6 A1
  constraint equal A0 A1
  constraint tangent L6 A2
  constraint tangent L5 A2
  constraint equal A0 A2
  constraint tangent L5 A3
  constraint tangent L4 A3
  constraint equal A0 A3
  measures "d207" distance of L5 L7
  measures "d208" distance of origin L5
  measures "d209" distance of L2 L6
  measures "d211" radius of A0
  measures "d212" distance of L0 L4
extrude "Extrude27" cut sketch "Sketch25" against normal blind 5 contours L4 L5 L6 L7 A0 A1 A2 A3
sketch "Sketch26" plane through (0, -14.3, 0) normal (0, 1, 0) x (-1, 0, 0)
  line L0 (55.628, 6.5) -> (-65.7592, 6.5)
  line L1 (-65.7592, 6.5) -> (-65.7592, 0)
  line L2 (-65.7592, 0) -> (55.628, 0)
  line L3 (55.628, 0) -> (55.628, 6.5)
  line L4 (-17.05, 4.5) -> (17.05, 4.5)
  line L5 (18.05, 3.5) -> (18.05, 3)
  line L6 (17.05, 2) -> (-17.05, 2)
  line L7 (-18.05, 3) -> (-18.05, 3.5)
  arc A0 (-17.05, 4.5) -> (-18.05, 3.5) centre (-17.05, 3.5) ccw
  arc A1 (18.05, 3.5) -> (17.05, 4.5) centre (17.05, 3.5) ccw
  arc A2 (17.05, 2) -> (18.05, 3) centre (17.05, 3) ccw
  arc A3 (-18.05, 3) -> (-17.05, 2) centre (-17.05, 3) ccw
  dimension "d227" = 2
  dimension "d228" = 2
  dimension "d229" = 36.1
  dimension "d230" = 18.05
  dimension "d231" = 1
  constraint horizontal L4
  constraint vertical L5
  constraint horizontal L6
  constraint vertical L7
  constraint tangent L7 A0
  constraint tangent L4 A0
  constraint tangent L4 A1
  constraint tangent L5 A1
  constraint equal A0 A1
  constraint tangent L5 A2
  constraint tangent L6 A2
  constraint equal A0 A2
  constraint tangent L6 A3
  constraint tangent L7 A3
  constraint equal A0 A3
  measures "d227" distance of L0 L4
  measures "d228" distance of L2 L6
  measures "d229" distance of L5 L7
  measures "d230" distance of origin L5
  measures "d231" radius of A0
extrude "Extrude28" cut sketch "Sketch26" against normal blind 5 contours L4 L5 L6 L7 A0 A1 A2 A3